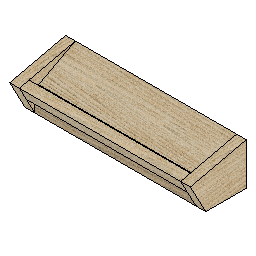
model (Autodesk Fusion 360 design; units mm, degrees)
Autodesk Fusion 360 part; units mm, degrees
sketch "Sketch1" plane through (0, 0, 0) normal (1, 0, 0) x (0, 1, 0)
  line L0 (0, 20) -> (10.6202, 0)
  line L1 (10.6202, 0) -> (85.9483, 40)
  line L2 (0, 0) -> (85.9483, 0) construction
  line L3 (85.9483, 0) -> (85.9483, 40) construction
  line L4 (0, 0) -> (0, 20) construction
  circle A0 centre (18.9045, 27.0439) radius 20 construction
  circle A1 centre (23.6902, 52.23) radius 40 construction
  circle A2 centre (23.9499, 75.0127) radius 60 construction
  line L5 (10.6202, 0) -> (10.6202, -20.3804) construction
  line L6 (10.6202, -38.3804) -> (85.9483, -38.3804)
  line L7 (85.9483, -38.3804) -> (85.9483, 40)
  line L8 (85.9483, 40) -> (85.9483, 160) construction
  line L9 (17.6858, 3.7519) -> (26.1276, -12.1457)
  line L10 (26.1276, -12.1457) -> (85.9483, 19.6196)
  line L11 (67.9483, 10.0615) -> (67.9483, -38.3804)
  line L12 (67.9483, -20.3804) -> (10.6202, -20.3804)
  line L13 (10.6202, -38.3804) -> (10.6202, -20.3804)
  line L14 (0, 20) -> (-18.139, 15.7791)
  line L15 (-18.139, 15.7791) -> (-5.2775, -8.4418)
  line L16 (-5.2775, -8.4418) -> (10.6202, 0)
  line L17 (-5.2775, -8.4418) -> (10.6202, -38.3804)
  line L18 (10.6202, -20.3804) -> (26.1276, -12.1457) construction
  line L19 (0, 20) -> (85.9483, 40)
  dimension "d2" = 20
  dimension "d3" = 40
  dimension "d4" = 40
  dimension "d5" = 80
  dimension "d6" = 120
  dimension "d9" = 120
  dimension "d11" = 18
  dimension "d13" = 18
  dimension "d14" = 18
  dimension "d17" = 27.969
  dimension "d18" = 8
  dimension "d19" = 18
  dimension "d20" = 62.031
  dimension "d21" = 57.3281
  dimension "d22" = 58
  dimension "d23" = 77.2897
  dimension "d24" = 75.131
  dimension "d25" = 27.4239
  constraint coincident L2.start L4.start
  constraint horizontal L2
  constraint vertical L3
  constraint coincident L0.end L2
  constraint perpendicular L0 L1
  constraint vertical L4
  constraint tangent L1 A0
  constraint tangent L1 A1
  constraint tangent L1 A2
  constraint tangent L0 A0
  constraint coincident L0.start A2
  constraint coincident L0.start A1
  constraint vertical L5
  constraint horizontal L6
  constraint vertical L7
  constraint vertical L8
  constraint coincident L1 L9.start
  constraint perpendicular L1 L9
  constraint coincident L3 L10.end
  constraint parallel L1 L10
  constraint coincident L10 L11.start
  constraint coincident L6 L11.end
  constraint vertical L11
  constraint coincident L11 L12.start
  constraint horizontal L12
  constraint perpendicular L12 L13
  constraint collinear L10 L18
  constraint collinear L15 L17
  constraint perpendicular L0 L16
  constraint perpendicular L15 L16
  constraint collinear L14 L19
  measures "d2" distance of L2.start L0.start
  measures "d3" distance of L1.end L2.end
  measures "d4" diameter of A0
  measures "d5" diameter of A1
  measures "d6" diameter of A2
  measures "d9" distance of L1.end L8.end
  measures "d11" distance of L9.start L9.end
  measures "d13" distance of L6.end L11
  measures "d14" distance of L11.end L12.start
  measures "d17" angle of L12 L18
  measures "d18" distance of L0.end L9.start
  measures "d19" distance of L0.end L15.end
  measures "d20" angle of L1 L3
  measures "d21" distance of L6.start L11.end
  measures "d22" distance of L6.end L10.end
  measures "d23" distance of L1.end L9.start
  measures "d24" angle of L14 L15
  measures "d25" distance of L14.end L15.end
extrude "Extrude1" add sketch "Sketch1" along normal blind 300 contours L1 L7 L9 L10 | L6 L11 L12 L13 makes body 1 at (100, 40.44, 15.8346) makes body 2 at (100, 29.7296, -38.3804)
extrude "Extrude2" add sketch "Sketch1" along normal blind 300 separate body contours L0 L14 L15 L16 | L6 L7 L10 L11 makes body 3 at (100, -13.8518, 7.7055) makes body 4 at (100, 85.9483, -19.047)
extrude "Extrude3" add sketch "Sketch1" against normal blind 18 separate body makes body 5
extrude "Extrude4" add sketch "Sketch1" along normal blind 18 from surface at 300 separate body makes body 6
equation "d9 = d6"
equation "th = 18 mm"
equation "d11 = th"
equation "d13 = th"
equation "d14 = th"
equation "d19 = th"
equation "d30 = -th"
equation "d33 = th"
